Autodesk Fusion 360 part; units mm, degrees
(part 2 of 2)
extrude "Extrude2" add sketch "Sketch3" against normal blind 15 contours S0 S1 S2 S3 S4 S5 S6 S7 S8 S9 L0 L1 S10 S11 S12 S13 S14 S15 S16 S17 S18 S19 S20 S21 S22 S23 S24 | S25 S26 S27 S28 S29 S30 S31 S32 S33 S34 S35 S36 S37 S38 S39 S40 S41 S42 S43 S44 S45 S46 S47 S48 S49 S50 S51 S52 L2 L3 S53 S54 S55 S56 S57 S58 S59 S60 S61 S62 S63 S64 S65 S66 L4 L5 S67 S68 S69 S70 S71 S72 S73 | S74 S75 S76 L6 L7 S77 S78 S79 S80 S81 S82 S83 S84 S85 S86 S87 S88 S89 S90 | S91 S92 S93 S94 S95 | S96 S97 S98 S99 S100 S101 S102 S103 S104 S105 S106 S107 S108 S109 S110 S111 S112 S113 S114 | S115 S116 S117 S118 L8 L9 S119 S120 S121 S122 S123 S124 S125 S126 S127 S128 S129 S130 S131 S132 S133 S134 S135 S136 S137 S138 | S139 S140 S141 | S142 S143 S144 S145 | S146 S147 S148 L10 L11 S149 S150 S151 S152 S153 S154 S155 S156 S157 S158 S159 S160 S161 S162 S163 S164 S165 S166 S167 S168 S169 S170 S171 S172 S173 S174 S175 S176 S177 S178 S179 | S180 S181 S182 S183 S184 S185 S186 S187 S188 S189 S190 S191 S192 S193 S194 S195 S196 S197 | S198 S199 S200 S201 S202 S203 S204 S205 S206 S207 S208 S209 S210 | S211 S212 S213 S214 S215 S216 S217 S218 S219 S220 S221 | S222 S223 L12 L13 S224 S225 S226 S227 S228 S229 S230 S231 S232 S233 S234 S235 S236 S237 S238 S239 S240 S241 S242 S243 S244 S245 S246 S247 S248 S249 S250 S251 S252 S253 S254 S255 S256 S257 S258 S259 S260 | S261 S262 S263 S264 S265 S266 S267 S268 S269 S270 S271 S272 S273 S274 S275 S276 | S277 S278 S279 S280 S281 S282 S283 S284 S285 S286 S287 S288 S289 | S290 S291 S292 S293 S294 S295 S296 S297 S298 S299 S300 S301 S302 | S303 S304 S305 S306 S307 S308 S309 S310 S311 S312 S313 S314 S315 S316 S317 L14 L15 S318 S319 S320 S321 S322 S323 S324 S325 S326 S327 S328 S329 S330 S331 S332 S333 S334 S335 S336 S337 S338 S339 S340 S341 S342 S343 S344 S345 S346 S347 S348 S349 S350 S351 S352 | L16 L17 L18 L19
extrude "Extrude3" add sketch "Sketch3" along normal blind 5 contours S0 S1 S2 S3 S4 S5 S6 S7 S8 S9 L0 L1 S10 S11 S12 S13 S14 S15 S16 S17 S18 S19 S20 S21 S22 S23 S24 | S25 S26 S27 S28 S29 S30 S31 S32 S33 S34 S35 S36 S37 S38 S39 S40 S41 S42 S43 S44 S45 S46 S47 S48 S49 S50 S51 S52 L2 L3 S53 S54 S55 S56 S57 S58 S59 S60 S61 S62 S63 S64 S65 S66 L4 L5 S67 S68 S69 S70 S71 S72 S73 | S74 S75 S76 L6 L7 S77 S78 S79 S80 S81 S82 S83 S84 S85 S86 S87 S88 S89 S90 | S91 S92 S93 S94 S95 | S96 S97 S98 S99 S100 S101 S102 S103 S104 S105 S106 S107 S108 S109 S110 S111 S112 S113 S114 | S115 S116 S117 S118 L8 L9 S119 S120 S121 S122 S123 S124 S125 S126 S127 S128 S129 S130 S131 S132 S133 S134 S135 S136 S137 S138 | S146 S147 S148 L10 L11 S149 S150 S151 S152 S153 S154 S155 S156 S157 S158 S159 S160 S161 S162 S163 S164 S165 S166 S167 S168 S169 S170 S171 S172 S173 S174 S175 S176 S177 S178 S179 | S222 S223 L12 L13 S224 S225 S226 S227 S228 S229 S230 S231 S232 S233 S234 S235 S236 S237 S238 S239 S240 S241 S242 S243 S244 S245 S246 S247 S248 S249 S250 S251 S252 S253 S254 S255 S256 S257 S258 S259 S260 | S303 S304 S305 S306 S307 S308 S309 S310 S311 S312 S313 S314 S315 S316 S317 L14 L15 S318 S319 S320 S321 S322 S323 S324 S325 S326 S327 S328 S329 S330 S331 S332 S333 S334 S335 S336 S337 S338 S339 S340 S341 S342 S343 S344 S345 S346 S347 S348 S349 S350 S351 S352
sketch "Sketch4" plane through (110.5079, 0, 67.6231) normal (0, 1, 0) x (1, 0, 0)
  line L0 (63.5387, -58.4266) -> (-70.5673, -58.4266)
  line L1 (-95.5673, -33.4266) -> (-95.5673, 8.1199)
  line L2 (-70.5673, 33.1199) -> (63.5387, 33.1199)
  line L3 (88.5387, 8.1199) -> (88.5387, -33.4266)
  line L4 (-127.9287, 79.9765) -> (125, 79.9765)
  line L5 (125, 79.9765) -> (125, -90)
  line L6 (125, -90) -> (-127.9287, -90)
  line L7 (-127.9287, -90) -> (-127.9287, 79.9765)
  arc A0 (-70.5673, 33.1199) -> (-95.5673, 8.1199) centre (-70.5673, 8.1199) ccw
  arc A1 (-95.5673, -33.4266) -> (-70.5673, -58.4266) centre (-70.5673, -33.4266) ccw
  arc A2 (88.5387, 8.1199) -> (63.5387, 33.1199) centre (63.5387, 8.1199) ccw
  arc A3 (63.5387, -58.4266) -> (88.5387, -33.4266) centre (63.5387, -33.4266) ccw
  dimension "d9" = 25
  constraint horizontal L0
  constraint vertical L1
  constraint horizontal L2
  constraint vertical L3
  constraint horizontal L4
  constraint vertical L5
  constraint horizontal L6
  constraint vertical L7
  constraint tangent L1 A0
  constraint tangent L2 A0
  constraint tangent L0 A1
  constraint tangent L1 A1
  constraint equal A0 A1
  constraint tangent L2 A2
  constraint tangent L3 A2
  constraint equal A0 A2
  constraint tangent L0 A3
  constraint tangent L3 A3
  constraint equal A0 A3
  measures "d9" radius of A0
extrude "Extrude4" cut sketch "Sketch4" against normal blind 25
